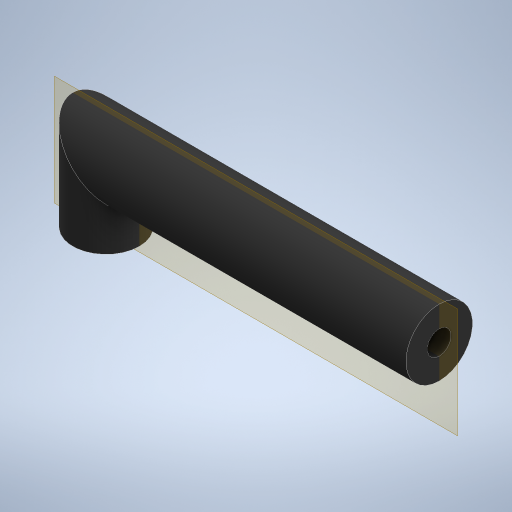
# Autodesk Inventor part: foam tube
Saved by Autodesk Inventor 2023 (Build 270158030, 158C)
## iProperties
Created: 2024-02-07
Part Number: foam tube
Material: Generisch
Document SubType Name: Modeling
Designer: Julian
Density: 1 g/cm^3
Appearance: Vorgabe
Author: Julian
Autodesk Inventor part; units mm, degrees
ref_plane "YZ Plane" through (0, 0, 0) normal (1, 0, 0) x (0, 1, 0)
ref_plane "XZ Plane" through (0, 0, 0) normal (0, 1, 0) x (-1, 0, 0)
sketch "Skizze1" plane through (0, 0, 0) normal (0, 1, 0) x (-1, 0, 0)
  circle A0 centre (0, 0) radius 14
  circle A1 centre (0, 0) radius 5
  dimension "d0" = 28
  dimension "d3" = 10
  constraints: 2 centre point, 2 coincident
  measures "d0" diameter of A0
  measures "d3" diameter of A1
sketch "Skizze2" plane through (0, 0, 0) normal (0, 0, 1) x (1, 0, 0)
  line L0 (0, 0) -> (0, 28)
  line L1 (0, 28) -> (140, 28)
  dimension "d1" = 28
  dimension "d2" = 140
  constraints: 4 end point, 1 horizontal, 1 vertical
  measures "d1" distance of L0.start L0.end
  measures "d2" distance of L0.end L1.end
sweep "Sweeping1" add profiles "Skizze1" path "Skizze2"
